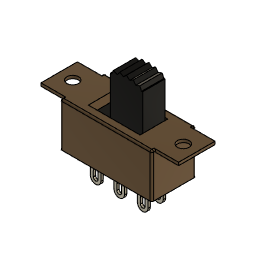
Diag_UP_PCB_v3 v24 (Autodesk Fusion 360 archive; units mm, degrees)
design "Slide_Switch_2"
Autodesk Fusion 360 part; units mm, degrees
sketch "switch" plane through (0, 0, 0) normal (0, 0, 1) x (1, 0, 0)
  line L0 (0, 0) -> (0, 16.8468) construction
  line L1 (-9.4, 0) -> (9.4, 0) construction
  circle A0 centre (-9.4, 0) radius 1
  circle A1 centre (9.4, 0) radius 1
  line L2 (7.8, -3.75) -> (-7.8, -3.75)
  line L3 (-7.8, -3.75) -> (-7.8, 3.75)
  line L4 (-7.8, 3.75) -> (7.8, 3.75)
  line L5 (7.8, 3.75) -> (7.8, -3.75)
  line L6 (7.8, -3.75) -> (-7.8, 3.75) construction
  line L7 (-7.8, -3.75) -> (7.8, 3.75) construction
  line L8 (-11.7, 3.1) -> (11.7, 3.1)
  line L9 (11.7, 3.1) -> (11.7, -3.1)
  line L10 (11.7, -3.1) -> (-11.7, -3.1)
  line L11 (-11.7, -3.1) -> (-11.7, 3.1)
  line L12 (-11.7, 3.1) -> (11.7, -3.1) construction
  line L13 (11.7, 3.1) -> (-11.7, -3.1) construction
  line L14 (4.4, -2.35) -> (-4.4, -2.35)
  line L15 (-4.4, -2.35) -> (-4.4, 2.35)
  line L16 (-4.4, 2.35) -> (4.4, 2.35)
  line L17 (4.4, 2.35) -> (4.4, -2.35)
  line L18 (4.4, -2.35) -> (-4.4, 2.35) construction
  line L19 (-4.4, -2.35) -> (4.4, 2.35) construction
  line L20 (4.4, 1.9) -> (-1.1, 1.9)
  line L21 (-1.1, 1.9) -> (-1.1, -1.9)
  line L22 (-1.1, -1.9) -> (4.4, -1.9)
  line L23 (4.4, -1.9) -> (4.4, 1.9)
  line L24 (4.4, 1.9) -> (-1.1, -1.9) construction
  line L25 (-1.1, 1.9) -> (4.4, -1.9) construction
  point P0 (1.65, 0)
  dimension "d1" = 2
  dimension "d2" = 2
  dimension "d3" = 18.8
  dimension "d4" = 7.5
  dimension "d6" = 15.6
  dimension "d7" = 23.4
  dimension "d8" = 6.2
  dimension "d9" = 8.8
  dimension "d10" = 4.7
  dimension "d11" = 5.5
  dimension "d12" = 3.8
  constraint coincident L0.start origin
  constraint vertical L0
  constraint horizontal L1
  constraint coincident L1.start A0.centre
  constraint coincident L1.end A1.centre
  constraint symmetric L0 A0 A1
  constraint horizontal L2
  constraint perpendicular L2 L3
  constraint parallel L2 L4
  constraint parallel L3 L5
  constraint coincident L6 L0.start
  constraint coincident L7 L0.start
  constraint horizontal L8
  constraint perpendicular L8 L9
  constraint parallel L8 L10
  constraint parallel L9 L11
  constraint coincident L12 L0.start
  constraint coincident L13 L0.start
  constraint horizontal L14
  constraint perpendicular L14 L15
  constraint parallel L14 L16
  constraint parallel L15 L17
  constraint coincident L18 L0.start
  constraint coincident L19 L0.start
  constraint horizontal L20
  constraint perpendicular L20 L21
  constraint parallel L20 L22
  constraint parallel L21 L23
  constraint coincident L24 P0
  constraint coincident L25 P0
  constraint coincident L1 P0
  constraint collinear L17 L23
  constraint coincident L0.start L1
  measures "d1" diameter of A0
  measures "d2" diameter of A1
  measures "d3" distance of L1.start L1.end
  measures "d4" distance of L2.end L3.end
  measures "d6" distance of L3 L5
  measures "d7" distance of L9.end L10.end
  measures "d8" distance of L8.end L9.end
  measures "d9" distance of L15.end L16.end
  measures "d10" distance of L14.end L15.end
  measures "d11" distance of L21.end L22.end
  measures "d12" distance of L20.end L21.end
extrude "Extrude1" add sketch "switch" against normal blind 7.5 contours L2 L3 L5 L10 | L3 L5 L8 L10 | L3 L4 L5 L8 | L14 L15 L16 L17 L20 L21 L22 | L17 L20 L21 L22 L23
extrude "Extrude2" add sketch "switch" against normal blind 0.5 contours L5 L8 L9 L10 | L3 L8 L10 L11
extrude "Extrude3" cut sketch "switch" against normal blind 1.5 contours L14 L15 L16 L17 L20 L21 L22
extrude "Extrude4" add sketch "switch" along normal blind 7.2 contours L17 L20 L21 L22 L23
sketch "profile" plane through (0, -1.9, 0) normal (0, -1, 0) x (1, 0, 0)
  line L0 (-1.1, 7.2) -> (-1.1, -1.5)
  line L1 (-1.1, -1.5) -> (4.4, -1.5)
  line L2 (4.4, -1.5) -> (4.4, 0)
  line L3 (4.4, 0) -> (4.4, 7.2)
  line L4 (4.4, 7.2) -> (-1.1, 7.2)
  line L5 (-1.1, 7.2) -> (-1.1, -1.5) construction
  line L6 (-1.1, 7.2) -> (4.4, 7.2) construction
  line L7 (4.4, 0) -> (4.4, 7.2) construction
  line L8 (1.65, 7.2) -> (1.65, -1.5) construction
  circle A0 centre (1.65, 1.2) radius 6 construction
  line L9 (1.65, 7.2) -> (1.1204, 6.7)
  line L10 (1.65, 7.2) -> (2.1796, 6.7)
  line L11 (1.1204, 6.7) -> (2.1796, 6.7) construction
  line L12 (1.1204, 6.7) -> (1.65, 1.2) construction
  line L13 (2.1796, 6.7) -> (1.65, 1.2) construction
  line L14 (-1.1, 6.5327) -> (1.65, 1.2) construction
  line L15 (1.65, 1.2) -> (4.4, 6.5327) construction
  line L16 (4.9178, 6.232) -> (4.2014, 6.1011)
  line L17 (4.9178, 6.232) -> (5.0897, 5.5243)
  line L18 (3.8976, 6.7631) -> (3.2193, 6.4979)
  line L19 (3.8976, 6.7631) -> (4.2014, 6.1011)
  line L20 (2.7949, 7.0898) -> (2.1796, 6.7)
  line L21 (2.7949, 7.0898) -> (3.2193, 6.4979)
  line L22 (0.5051, 7.0898) -> (0.0807, 6.4979)
  line L23 (0.5051, 7.0898) -> (1.1204, 6.7)
  line L24 (-0.5976, 6.7631) -> (-0.9014, 6.1011)
  line L25 (-0.5976, 6.7631) -> (0.0807, 6.4979)
  line L26 (-1.6178, 6.232) -> (-1.7897, 5.5243)
  line L27 (-1.6178, 6.232) -> (-0.9014, 6.1011)
  line L28 (-1.1, 7.2) -> (-1.1, 6.1374)
  line L29 (-1.1, 7.2) -> (4.4, 7.2)
  line L30 (4.4, 7.2) -> (4.4, 6.1374)
  dimension "d21" = 12
  dimension "d23" = 0.5
  dimension "d24" = 11
  dimension "d26" = 66
  constraint midpoint L6 L8.start
  constraint midpoint L1 L8.end
  constraint coincident L8 A0.centre
  constraint tangent L6 A0
  constraint symmetric L9.start L8 L10.start
  constraint symmetric L8 L9.end L10.end
  constraint horizontal L11
  constraint coincident A0.centre L12.end
  constraint coincident L0 L14.start
  constraint coincident A0 L14.start
  constraint coincident L3 L15.end
  constraint coincident A0 L15.end
  constraint coincident L0.start L4.end
  constraint coincident L0 L28.end
  constraint coincident L27 L28.end
  constraint coincident L3.end L4.start
  constraint coincident L7 L30.end
  constraint coincident L16 L30.end
  measures "d21" diameter of A0
  measures "d23" distance of L4 L11
  measures "d24" angle of L12 L13
extrude "Extrude5" cut sketch "profile" against normal blind 4 contours L0 L4 L9 L22 L23 L24 L25 L27 L28 L29 | L3 L4 L10 L16 L18 L19 L20 L21 L29 L30
sketch "contacts" plane through (0, 0, -7.5) normal (0, 0, -1) x (1, 0, 0)
  line L0 (-7.8, -3.75) -> (7.8, -3.75)
  line L1 (7.8, -3.75) -> (7.8, 3.75)
  line L2 (7.8, 3.75) -> (-7.8, 3.75)
  line L3 (-7.8, 3.75) -> (-7.8, -3.75)
  line L4 (-7.8, 3.75) -> (-7.8, -3.75) construction
  line L5 (7.8, 3.75) -> (-7.8, 3.75) construction
  line L6 (7.8, -3.75) -> (7.8, 3.75) construction
  line L7 (-7.8, -3.75) -> (7.8, -3.75) construction
  line L8 (-7.8, 0) -> (7.8, 0) construction
  line L9 (0, 3.75) -> (0, -3.75) construction
  line L10 (-0.9, 1.1) -> (0.9, 1.1)
  line L11 (0.9, 1.1) -> (0.9, 1.5)
  line L12 (0.9, 1.5) -> (-0.9, 1.5)
  line L13 (-0.9, 1.5) -> (-0.9, 1.1)
  line L14 (-4.9, 1.1) -> (-3.1, 1.1)
  line L15 (-3.1, 1.1) -> (-3.1, 1.5)
  line L16 (-3.1, 1.5) -> (-4.9, 1.5)
  line L17 (-4.9, 1.5) -> (-4.9, 1.1)
  line L18 (3.1, 1.5) -> (4.9, 1.5)
  line L19 (3.1, 1.1) -> (3.1, 1.5)
  line L20 (4.9, 1.1) -> (3.1, 1.1)
  line L21 (4.9, 1.5) -> (4.9, 1.1)
  line L22 (3.1, -1.1) -> (3.1, -1.5)
  line L23 (-4.9, -1.1) -> (-3.1, -1.1)
  line L24 (-0.9, -1.1) -> (0.9, -1.1)
  line L25 (4.9, -1.1) -> (3.1, -1.1)
  line L26 (0.9, -1.5) -> (-0.9, -1.5)
  line L27 (-4.9, -1.5) -> (-4.9, -1.1)
  line L28 (0.9, -1.1) -> (0.9, -1.5)
  line L29 (-0.9, -1.5) -> (-0.9, -1.1)
  line L30 (-3.1, -1.1) -> (-3.1, -1.5)
  line L31 (-3.1, -1.5) -> (-4.9, -1.5)
  line L32 (3.1, -1.5) -> (4.9, -1.5)
  line L33 (4.9, -1.5) -> (4.9, -1.1)
  dimension "d29" = 0.4
  dimension "d30" = 1.8
  dimension "d31" = 0.4
  dimension "d32" = 1.8
  dimension "d33" = 9.8
  dimension "d34" = 3
  constraint midpoint L4 L8.start
  constraint midpoint L6 L8.end
  constraint midpoint L5 L9.start
  constraint midpoint L7 L9.end
  constraint horizontal L10
  constraint vertical L11
  constraint horizontal L12
  constraint vertical L13
  constraint symmetric L9 L11 L13
  constraint horizontal L14
  constraint vertical L15
  constraint horizontal L16
  constraint vertical L17
  constraint collinear L10 L14
  constraint symmetric L9 L14.start L20.start
  constraint symmetric L9 L14.end L19.start
  constraint symmetric L9 L15.end L18.start
  constraint symmetric L9 L16.end L18.end
  constraint symmetric L8 L10.start L24.start
  constraint symmetric L8 L10.end L24.end
  constraint symmetric L8 L11.end L26.start
  constraint symmetric L8 L12.end L26.end
  constraint symmetric L8 L14.start L23.start
  constraint symmetric L8 L14.end L23.end
  constraint symmetric L8 L15.end L30.end
  constraint symmetric L8 L16.end L27.start
  constraint symmetric L8 L18.start L22.end
  constraint symmetric L8 L18.end L32.end
  constraint symmetric L8 L19.start L22.start
  constraint symmetric L8 L20.start L25.start
  measures "d29" distance of L10 L12
  measures "d30" distance of L11 L13
  measures "d31" distance of L14 L16
  measures "d32" distance of L15 L17
  measures "d33" distance of L17 L21
  measures "d34" distance of L18 L32
extrude "Extrude6" add sketch "contacts" along normal blind 4.4 contours L10 L11 L12 L13 | L14 L15 L16 L17 | L18 L19 L20 L21 | L22 L25 L32 L33 | L23 L27 L30 L31 | L24 L26 L28 L29
fillet "Fillet1" radius 0.9 12 edges at (-3.1, -1.3, -11.9) (-4.9, -1.3, -11.9) (-3.1, 1.3, -11.9) (-4.9, 1.3, -11.9) (-0.9, 1.3, -11.9) (0.9, 1.3, -11.9) (-0.9, -1.3, -11.9) (0.9, -1.3, -11.9) (3.1, -1.3, -11.9) (3.1, 1.3, -11.9) (4.9, 1.3, -11.9) (4.9, -1.3, -11.9)
sketch "Sketch4" plane through (0, 1.5, 0) normal (0, 1, 0) x (-1, 0, 0)
  arc A0 (-0.9, -11) -> (0.9, -11) centre (0, -11) ccw
  line L0 (0.9, -11) -> (0.9, -7.5)
  line L1 (0.9, -7.5) -> (-0.9, -7.5)
  line L2 (-0.9, -7.5) -> (-0.9, -11)
  arc A1 (-4.9, -11) -> (-3.1, -11) centre (-4, -11) ccw construction
  arc A2 (-0.9, -11) -> (0.9, -11) centre (0, -11) ccw construction
  arc A3 (3.1, -11) -> (4.9, -11) centre (4, -11) ccw construction
  line L3 (-4.9, -11) -> (-3.1, -11) construction
  circle A4 centre (-4, -11) radius 0.4
  line L4 (-4, -11) -> (-4, -10) construction
  circle A5 centre (-4, -10) radius 0.4
  line L5 (-4, -10) -> (-3.6, -10) construction
  line L6 (-4, -10) -> (-4.4, -10) construction
  line L7 (-3.6, -10) -> (-3.6, -11)
  line L8 (-4.4, -10) -> (-4.4, -11)
  line L9 (7.8, -7.5, 2.25) -> (-7.8, -7.5, 2.25) construction
  line L10 (-4, -11.9) -> (0, -11.9) construction
  line L11 (-2, -11.9) -> (-2, -7.5511) construction
  circle A6 centre (0, -10) radius 0.4
  circle A7 centre (0, -11) radius 0.4
  line L12 (-0.4, -10) -> (-0.4, -11)
  line L13 (0.4, -10) -> (0.4, -11)
  line L14 (0, -11.9) -> (0, -8.0759) construction
  circle A8 centre (4, -10) radius 0.4
  line L15 (4.4, -10) -> (4.4, -11)
  circle A9 centre (4, -11) radius 0.4
  line L16 (3.6, -10) -> (3.6, -11)
  dimension "d39" = 0.8
  dimension "d40" = 1
  dimension "d41" = 0.8
  constraint coincident A1.start L3.start
  constraint coincident A1.end L3.end
  constraint concentric A1 A4
  constraint coincident A1.centre A4.centre
  constraint perpendicular L3 L4
  constraint coincident L4.end A5.centre
  constraint coincident A5 L5.end
  constraint perpendicular L4 L5
  constraint coincident A5 L6.end
  constraint perpendicular L4 L6
  constraint coincident A4 L7.end
  constraint coincident L3 L7.end
  constraint coincident A4 L8.end
  constraint coincident L3 L8.end
  constraint midpoint A0 L10.end
  constraint midpoint A1 L10.start
  constraint midpoint L10 L11.start
  constraint perpendicular L10 L11
  constraint symmetric A4 L11 A7
  constraint symmetric A5 L11 A6
  constraint symmetric L5.end L11 L12.start
  constraint symmetric L6.end L11 L13.start
  constraint symmetric L7.end L11 L12.end
  constraint symmetric L8.end L11 L13.end
  constraint perpendicular L1 L14
  constraint symmetric A4 L14 A9
  constraint symmetric A5 L14 A8
  constraint symmetric L5.end L14 L16.start
  constraint symmetric L6.end L14 L15.start
  constraint symmetric L7.end L14 L16.end
  constraint symmetric L8.end L14 L15.end
  measures "d39" diameter of A4
  measures "d40" distance of A1.centre L4.end
  measures "d41" diameter of A5
extrude "Extrude7" cut sketch "Sketch4" against normal blind 3.1 contours A4 | A4 A5 L7 L8 | A5 | A6 | A6 A7 L12 L13 | A7 | A8 | A8 L15 A9 L16 | A9
fillet "Fillet2" radius 0.3 4 edges at (7.8, 3.75, -3.75) (7.8, -3.75, -3.75) (-7.8, 3.75, -3.75) (-7.8, -3.75, -3.75)
fillet "Fillet3" radius 0.3 10 edges at (-7.8, 3.275, 0) (-7.7121, 3.6621, 0) (0, 3.75, 0) (7.7121, 3.6621, 0) (7.8, 3.275, 0) (7.8, -3.275, 0) (7.7121, -3.6621, 0) (0, -3.75, 0) (-7.7121, -3.6621, 0) (-7.8, -3.275, 0)
equation "d2 = d1"
equation "d31 = d29"
equation "d32 = d30"
equation "d41 = d39"
